Test arbre moteur (Autodesk Fusion 360 design; units mm, degrees)
Autodesk Fusion 360 part; units mm, degrees
note: some values were not read from the file. Set by a fixed rule: which sketch regions a step uses.
sketch "Sketch1" plane through (0, 0, 0) normal (0, 0, 1) x (1, 0, 0)
  circle A0 centre (0, 0) radius 3.1
  line L0 (-1.833, -2.5) -> (1.833, -2.5)
  line L1 (-3, -3.1) -> (0, -3.1) construction
  circle A1 centre (0, 0) radius 7.5
  dimension "d1" = 6.2
  dimension "d2" = 0.6
  dimension "d3" = 15
  constraint coincident A0.centre A1.centre
  constraint coincident A0 L0.start
  constraint coincident A0 L0.end
  constraint horizontal L0
  constraint horizontal L1
  constraint coincident A0 L1.end
  constraint tangent A0 L1
  measures "d1" diameter of A0
  measures "d2" distance of L0 L1
  measures "d3" diameter of A1
extrude "Extrude1" add sketch "Sketch1" along normal blind 0.5 contours A0 L0 | A0 L0
extrude "Extrude2" add sketch "Sketch1" along normal blind 10 contours A0 L0 | A1 picked at (0.4882, -2.5774)
